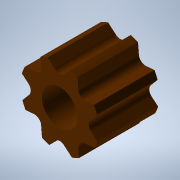
# Autodesk Inventor part: MSF-25 Sleeve
Saved by Autodesk Inventor 2021 (Build 250183000, 183)
## iProperties
Created: 2026-05-20
Part Number: MSF-25 Sleeve
Material: Generic
Catalog Web Link: www.3dfindit.com
Description: MSF mid-MSF
Vendor: NBK
Document SubType Name: Modeling
Designer: psAdmin
Manufacturer: NBK
Mass: 3.57864 g
Surface Area: 23.675 cm^2
Volume: 3.57864 cm^3
Density: 1 g/cm^3
Appearance: PSOLRGB-224-162-31
Category: PARTsolutions
Company: NBK
Title: MSF-25
Author: Cadenas PARTsolutions
Comments: MSF
PSOL_IDENT_0: {$CADENAS_DATA/23d-libs/nbk/motion_control_parts/couplicon_mini/msf/msf_middle.prj},151 {VTYP=3D},{N
PSOL_IDENT_1: B=MSF-25 Sleeve},{LINA=MSF-25},{NN=MSF mid},{DATE=08.05.2026 02:12:20},{GEOMDATE=07.07.2008},{VERSIO
PSOL_IDENT_2: N=},{LINEID=40},{WBVAR=},{WBNUMERIC=}  {NB=MSF-25 Sleeve},{LINA=MSF-25},{KT=DUMMY},{CN=MSF-25},{A=25
PSOL_IDENT_3: },{B=18},{L=12},{W=41},{F=6},{M=M4},{WT=1.7},{C=17},{K=22},{D=10/10},{NDM=4.000},{KDM=2.91746},{P=1.
PSOL_IDENT_4: 000},{K1=3.760},{DU=16.250},{DL=10.000},{DR=10.000},{CLR=0.878,0.635,0.122,0.00}
NB: MSF-25 Sleeve
NN: MSF mid
NT: MSF
NBSYN: $CN. Sleeve
LINA: MSF-25
CATALOG: NBK (Nabeya Bi-tech Kaisha
CN: MSF-25
A: 25
B: 18
L: 12
W: 41
F: 6
M: M4
WT: 1.7
C: 17
K: 22
D: 10/10
NDM: 4
P: 1
K1: 3.76
DU: 16.25
DL: 10
DR: 10
CLR: 0.878,0.635,0.122,0.00
SUPPLIER: NBK
ARTICLENO: MSF-25 Sleeve
BOMINFO: MSF-25
CREATOR: CADENAS GmbH
Autodesk Inventor part; units mm, degrees
sketch "Sketch_1" plane through (0, 0, 0) normal (0, 0, 1) x (1, 0, 0)
  line L0 (-10.597, 2.9503) -> (-8.764, 1.4122)
  arc A0 (-8.764, -1.4122) -> (-8.764, 1.4122) centre (-10.005, 0) ccw
  line L1 (-8.764, -1.4122) -> (-10.4531, -3.4252)
  arc A1 (-10.4531, -3.4252) -> (-9.5793, -5.4071) centre (0, 0) ccw
  line L2 (-9.5793, -5.4071) -> (-7.1956, -5.1985)
  arc A2 (-5.1985, -7.1956) -> (-7.1956, -5.1985) centre (-7.0746, -7.0746) ccw
  line L3 (-5.1985, -7.1956) -> (-4.9695, -9.8135)
  arc A3 (-4.9695, -9.8135) -> (-2.9503, -10.597) centre (0, 0) ccw
  line L4 (-2.9503, -10.597) -> (-1.4122, -8.764)
  arc A4 (1.4122, -8.764) -> (-1.4122, -8.764) centre (0, -10.005) ccw
  line L5 (1.4122, -8.764) -> (3.4252, -10.4531)
  arc A5 (3.4252, -10.4531) -> (5.4071, -9.5793) centre (0, 0) ccw
  line L6 (5.4071, -9.5793) -> (5.1985, -7.1956)
  arc A6 (7.1956, -5.1985) -> (5.1985, -7.1956) centre (7.0746, -7.0746) ccw
  line L7 (7.1956, -5.1985) -> (9.8135, -4.9695)
  arc A7 (9.8135, -4.9695) -> (10.597, -2.9503) centre (0, 0) ccw
  line L8 (10.597, -2.9503) -> (8.764, -1.4122)
  arc A8 (8.764, 1.4122) -> (8.764, -1.4122) centre (10.005, 0) ccw
  line L9 (8.764, 1.4122) -> (10.4531, 3.4252)
  arc A9 (10.4531, 3.4252) -> (9.5793, 5.4071) centre (0, 0) ccw
  line L10 (9.5793, 5.4071) -> (7.1956, 5.1985)
  arc A10 (5.1985, 7.1956) -> (7.1956, 5.1985) centre (7.0746, 7.0746) ccw
  line L11 (5.1985, 7.1956) -> (4.9695, 9.8135)
  arc A11 (4.9695, 9.8135) -> (2.9503, 10.597) centre (0, 0) ccw
  line L12 (2.9503, 10.597) -> (1.4122, 8.764)
  arc A12 (-1.4122, 8.764) -> (1.4122, 8.764) centre (0, 10.005) ccw
  line L13 (-1.4122, 8.764) -> (-3.4252, 10.4531)
  arc A13 (-3.4252, 10.4531) -> (-5.4071, 9.5793) centre (0, 0) ccw
  line L14 (-5.4071, 9.5793) -> (-5.1985, 7.1956)
  arc A14 (-7.1956, 5.1985) -> (-5.1985, 7.1956) centre (-7.0746, 7.0746) ccw
  line L15 (-7.1956, 5.1985) -> (-9.8135, 4.9695)
  arc A15 (-9.8135, 4.9695) -> (-10.597, 2.9503) centre (0, 0) ccw
  constraints: 32 end point, 32 point on circle, 16 centre point
extrude "Extrusion1" add sketch "Sketch_1" along normal blind 17
sketch "Sketch2" plane through (0, 0, 0) normal (0, 0, -1) x (-1, 0, 0)
  point P0 (0, 0)
hole "Hole1" at (0, 0, 0) direction (0, 0, 1) diameter 10 depth 17
ref_plane "left_XY" through (0, 0, 0) normal (0, 0, 1) x (1, 0, 0)
ref_plane "left_YZ" through (0, 0, 0) normal (1, 0, 0) x (0, 1, 0)
ref_plane "left_ZX" through (0, 0, 0) normal (0, 1, 0) x (0, 0, 1)
ref_plane "right_XY" through (0, 0, 17) normal (0, 0, 1) x (1, 0, 0)
ref_plane "right_YZ" through (0, 0, 17) normal (1, 0, 0) x (0, 1, 0)
ref_plane "right_ZX" through (0, 0, 17) normal (0, 1, 0) x (0, 0, 1)
body "Solid1"
